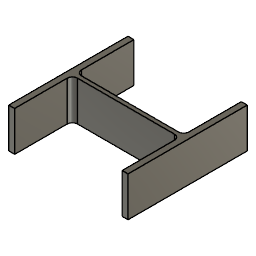
H-300×300×10×15 (Autodesk Fusion 360 design; units mm, degrees)
Autodesk Fusion 360 part; units mm, degrees
sketch "スケッチ1" plane through (0, 0, 0) normal (0, 0, 1) x (1, 0, 0)
  line L0 (0, 150) -> (0, -150)
  line L1 (300, -150) -> (300, 150)
  line L2 (285, -18) -> (285, -150)
  line L3 (15, -150) -> (15, -18)
  line L4 (0, -150) -> (15, -150)
  line L5 (285, -150) -> (300, -150)
  line L6 (15, 18) -> (15, 150)
  line L7 (285, 150) -> (285, 18)
  line L8 (272, 5) -> (28, 5)
  line L9 (28, -5) -> (272, -5)
  line L10 (15, 150) -> (0, 150)
  line L11 (300, 150) -> (285, 150)
  arc A0 (28, -5) -> (15, -18) centre (28, -18) ccw
  arc A1 (15, 18) -> (28, 5) centre (28, 18) ccw
  arc A2 (272, 5) -> (285, 18) centre (272, 18) ccw
  arc A3 (285, -18) -> (272, -5) centre (272, -18) ccw
extrude "押し出し1" add sketch "スケッチ1" along normal blind 100
